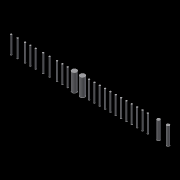
# Autodesk Inventor part: 3d_Welding_Tooling - Bot Wire
Saved by Autodesk Inventor 2018.3 (Build 223284000, 284)
## iProperties
Created: 2026-01-22
Part Number: 3d_Welding_Tooling - Bot Wire
Material: Genérico
Document SubType Name: Modeling
Designer: aca6
Density: 1 g/cm^3
Appearance: Valor por defecto
Author: aca6
Autodesk Inventor part; units mm, degrees
ref_plane "YZ Plane" through (0, 0, 0) normal (1, 0, 0) x (0, 1, 0)
ref_plane "XZ Plane" through (0, 0, 0) normal (0, 1, 0) x (-1, 0, 0)
ref_plane "XY Plane" through (0, 0, 0) normal (0, 0, 1) x (1, 0, 0)
sketch "Sketch1" plane through (0, 0, 0) normal (0, 0, 1) x (1, 0, 0)
  line L0 (21.2149, 0) -> (-24.25, 0) construction
  circle A0 centre (20.25, 0) radius 0.405
  circle A1 centre (17.55, 0) radius 0.405
  circle A2 centre (15, 0) radius 0.2025
  circle A3 centre (13.5, 0) radius 0.2025
  circle A4 centre (12, 0) radius 0.2025
  circle A5 centre (10.5, 0) radius 0.2025
  circle A6 centre (9, 0) radius 0.2025
  circle A7 centre (7.5, 0) radius 0.2025
  circle A8 centre (6, 0) radius 0.2025
  circle A9 centre (4.5, 0) radius 0.2025
  circle A10 centre (3, 0) radius 0.2025
  circle A11 centre (1.5, 0) radius 0.2025
  circle A12 centre (0, 0) radius 0.2025
  circle A13 centre (-1.5, 0) radius 0.2025
  circle A14 centre (-7.5, 0) radius 0.2025
  circle A15 centre (-9, 0) radius 0.2025
  circle A16 centre (-10.5, 0) radius 0.2025
  circle A17 centre (-12.6, 0) radius 0.2025
  circle A18 centre (-14.4, 0) radius 0.2025
  circle A19 centre (-16.5, 0) radius 0.2025
  circle A20 centre (-18, 0) radius 0.2025
  circle A21 centre (-19.5, 0) radius 0.2025
  circle A22 centre (-21.6, 0) radius 0.2025
  circle A23 centre (-23.4, 0) radius 0.2025
  line L1 (-25.25, -2) -> (-25.25, -0.4) projected
  arc A24 (-4.96, 0) -> (-6.33, 0) centre (-5.645, 0) ccw projected
  arc A25 (-6.33, 0) -> (-4.96, 0) centre (-5.645, 0) ccw projected
  arc A26 (-4.04, 0) -> (-2.67, 0) centre (-3.355, 0) ccw projected
  arc A27 (-2.67, 0) -> (-4.04, 0) centre (-3.355, 0) ccw projected
  point P0 (0, 0)
  dimension "d0" = 0.81
  dimension "d1" = 0.81
  dimension "d2" = 0.405
  dimension "d3" = 0.405
  dimension "d4" = 0.405
  dimension "d5" = 0.405
  dimension "d6" = 0.405
  dimension "d7" = 0.405
  dimension "d8" = 0.405
  dimension "d9" = 0.405
  dimension "d10" = 0.405
  dimension "d11" = 0.405
  dimension "d12" = 0.405
  dimension "d13" = 0.405
  dimension "d14" = 0.405
  dimension "d15" = 0.405
  dimension "d16" = 0.405
  dimension "d17" = 0.405
  dimension "d18" = 0.405
  dimension "d19" = 0.405
  dimension "d20" = 0.405
  dimension "d21" = 0.405
  dimension "d22" = 0.405
  dimension "d23" = 0.405
  dimension "d24" = 1.85
  dimension "d25" = 1.8
  dimension "d26" = 2.1
  dimension "d27" = 1.5
  dimension "d28" = 2.1
  dimension "d29" = 1.8
  dimension "d30" = 2.1
  dimension "d31" = 1.5
  dimension "d32" = 1.5
  dimension "d33" = 6
  dimension "d34" = 1.5
  dimension "d35" = 1.5
  dimension "d36" = 1.5
  dimension "d37" = 1.5
  dimension "d38" = 1.5
  dimension "d39" = 1.5
  dimension "d40" = 1.5
  dimension "d44" = 2.7
  dimension "d46" = 2.55
  constraints: 24 centre point, 6 coincident, 21 other
  measures "d0" diameter of A0
  measures "d1" diameter of A1
  measures "d2" diameter of A2
  measures "d3" diameter of A3
  measures "d4" diameter of A4
  measures "d5" diameter of A5
  measures "d6" diameter of A6
  measures "d7" diameter of A7
  measures "d8" diameter of A8
  measures "d9" diameter of A9
  measures "d10" diameter of A10
  measures "d11" diameter of A11
  measures "d12" diameter of A12
  measures "d13" diameter of A13
  measures "d14" diameter of A14
  measures "d15" diameter of A15
  measures "d16" diameter of A16
  measures "d17" diameter of A17
  measures "d18" diameter of A18
  measures "d19" diameter of A19
  measures "d20" diameter of A20
  measures "d21" diameter of A21
  measures "d22" diameter of A22
  measures "d23" diameter of A23
  measures "d24" distance from line of L1 A23.centre
  measures "d25" distance of A22.centre A23.centre
  measures "d26" distance of A21.centre A22.centre
  measures "d27" distance of A19.centre point (-18, 0)
  measures "d28" distance of A18.centre A19.centre
  measures "d29" distance of A17.centre A18.centre
  measures "d30" distance of A16.centre A17.centre
  measures "d31" distance of A16.centre point (-9, 0)
  measures "d32" distance of A14.centre point (-9, 0)
  measures "d33" distance of A14.centre A13.centre
  measures "d34" distance of point (0, 0) A11.centre
  measures "d35" distance of A10.centre A11.centre
  measures "d36" distance of point (4.5, 0) A8.centre
  measures "d37" distance of A7.centre A8.centre
  measures "d38" distance of point (9, 0) A5.centre
  measures "d39" distance of A4.centre A5.centre
  measures "d40" distance of point (13.5, 0) A2.centre
  measures "d44" distance of A0.centre A1.centre
  measures "d46" distance of A1.centre A2.centre
extrude "Extrusion1" add sketch "Sketch1" along normal blind 5
body "Solid1"
